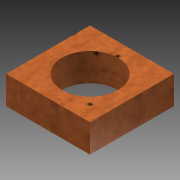
# Autodesk Inventor part: Dershatel_Motora
Saved by Autodesk Inventor 2015 (Build 190159000, 159)
## iProperties
Created: 2016-05-09
Part Number: Dershatel_Motora
Material: Wood (Cherry)
Document SubType Name: Modeling
Designer: Andreas
Density: 0.63 g/cm^3
Appearance: Cherry - Natural Low Gloss
Author: Andreas
Autodesk Inventor part; units mm, degrees
ref_plane "YZ Plane" through (0, 0, 0) normal (1, 0, 0) x (0, 1, 0)
ref_plane "XZ Plane" through (0, 0, 0) normal (0, 1, 0) x (-1, 0, 0)
ref_plane "XY Plane" through (0, 0, 0) normal (0, 0, 1) x (1, 0, 0)
sketch "Sketch1" plane through (0, 0, 0) normal (0, 0, 1) x (1, 0, 0)
  line L0 (0, 0) -> (30, 0)
  line L1 (30, 0) -> (30, -30)
  line L2 (30, -30) -> (0, -30)
  line L3 (0, -30) -> (0, 0)
  circle A0 centre (15, -15) radius 10
  point P0 (15, -30)
  point P1 (0, -15)
  dimension "d0" = 30
  dimension "d1" = 30
  dimension "d2" = 20
  constraints: 8 end point, 3 perpendicular, 2 midpoint, 1 centre point, 1 horizontal, 1 horizontal alignment, 1 vertical alignment
  measures "d0" distance of L0.start L0.end
  measures "d1" distance of L0.end L1.end
  measures "d2" diameter of A0
extrude "Extrusion1" add sketch "Sketch1" along normal blind 10
body "Solid1"
